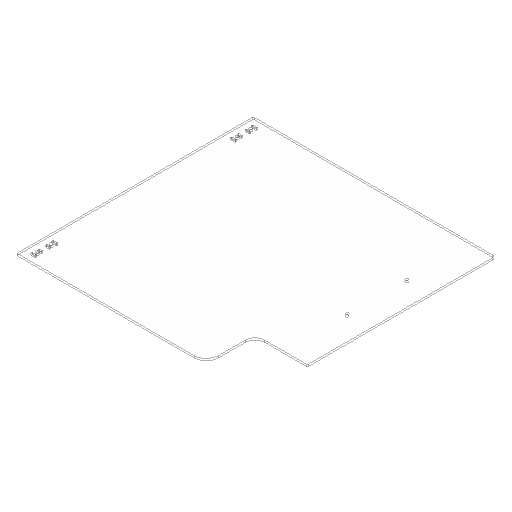
# Autodesk Inventor part: LC_PLEXI_4mm_Front_Door
Saved by Autodesk Inventor 2026.1 (Build 301233000, 233)
## iProperties
Created: 2016-06-27
Part Number: LC_PLEXI_4mm_Front_Door
Material: Ogólny
Document SubType Name: Modeling
Designer: Andrzej
Density: 1 g/cm^3
Appearance: Przezroczysty - jasny
Mass: 916.961 g
Surface Area: 4666.78 cm^2
Volume: 916.961 cm^3
Author: Andrzej
Autodesk Inventor part; units mm, degrees
ref_plane "YZ Plane" through (0, 0, 0) normal (1, 0, 0) x (0, 1, 0)
ref_plane "XZ Plane" through (0, 0, 0) normal (0, 1, 0) x (-1, 0, 0)
ref_plane "XY Plane" through (0, 0, 0) normal (0, 0, 1) x (1, 0, 0)
sketch "Szkic1" plane through (0, 0, 0) normal (0, 0, 1) x (1, 0, 0)
  line L0 (-549.5887, -180.0814) -> (-549.5887, 304.9186)
  line L1 (-549.5887, 304.9186) -> (-53.5887, 304.9186)
  line L2 (-53.5887, 304.9186) -> (-53.5887, -80.0814)
  line L3 (-53.5887, -80.0814) -> (-141.0887, -80.0814)
  line L4 (-161.0887, -100.0814) -> (-161.0887, -155.0814)
  line L5 (-186.0887, -180.0814) -> (-549.5887, -180.0814)
  arc A0 (-141.0887, -80.0814) -> (-161.0887, -100.0814) centre (-141.0887, -100.0814) ccw
  arc A1 (-186.0887, -180.0814) -> (-161.0887, -155.0814) centre (-186.0887, -155.0814) ccw
  point P0 (0, 0)
  point P1 (-161.0887, -80.0814)
  point P2 (-161.0887, -180.0814)
  point P3 (-531.0887, 281.4186)
  point P4 (-531.0887, 253.4186)
  point P5 (-531.0887, -128.5814)
  point P6 (-531.0887, -156.5814)
  point P7 (-103.5887, 173.4186)
  point P8 (-103.5887, 51.4186)
  dimension "d0" = 485
  dimension "d1" = 496
  dimension "d2" = 107.5
  dimension "d3" = 100
  dimension "d6" = 20
  dimension "d7" = 25
  dimension "d8" = 28
  dimension "d9" = 23.5
  dimension "d11" = 28
  dimension "d12" = 23.5
  dimension "d13" = 18.5
  dimension "d14" = 18.5
  dimension "d17" = 18.5
  dimension "d18" = 18.5
  dimension "d31" = 385
  dimension "d32" = 122
  dimension "d33" = 131.5
  dimension "d34" = 50
  dimension "d35" = 50
  constraints: 12 end point, 5 perpendicular, 4 point on circle, 4 point on line, 4 tangent, 2 centre point, 1 vertical
  measures "d0" distance of L0.start L0.end
  measures "d1" distance of L0.end L1.end
  measures "d2" distance between parallel lines of L2 L4
  measures "d3" distance between parallel lines of L5 L3
  measures "d6" radius of A0
  measures "d7" radius of A1
  measures "d8" distance of point (-531.089, 281.419) point (-531.089, 253.419)
  measures "d9" distance from line of L1 point (-531.089, 281.419)
  measures "d11" distance of point (-531.089, -156.581) point (-531.089, -128.581)
  measures "d12" distance from line of L5 point (-531.089, -156.581)
  measures "d13" distance from line of L0 point (-531.089, 281.419)
  measures "d14" distance from line of L0 point (-531.089, 253.419)
  measures "d17" distance from line of L0 point (-531.089, -128.581)
  measures "d18" distance from line of L0 point (-531.089, -156.581)
  measures "d31" distance of L1.end L2.end
  measures "d32" distance of point (-103.589, 173.419) point (-103.589, 51.419)
  measures "d33" distance from line of point (-103.589, 173.419) L1
  measures "d34" distance from line of L2 point (-103.589, 173.419)
  measures "d35" distance from line of L2 point (-103.589, 51.419)
extrude "Wyciągnięcie proste1" add sketch "Szkic1" along normal blind 4
hole "Otwór1" at (-531.0887, 281.4186, 0) at (-531.0887, 253.4186, 0) at (-531.0887, -128.5814, 0) at (-531.0887, -156.5814, 0) direction (0, 0, 1) diameter 6 end through all
fillet "Zaokrąglenie2" radius 2 2 edges at (-53.5887, -80.0814, 2) (-549.5887, -180.0814, 2)
fillet "Zaokrąglenie2" radius 2 1 edges at (-549.5887, 304.9186, 2)
fillet "Zaokrąglenie2" radius 5 1 edges at (-53.5887, 304.9186, 2)
hole "Otwór2" at (-103.5887, 173.4186, 0) at (-103.5887, 51.4186, 0) direction (0, 0, 1) diameter 6 end through all
sketch "Szkic2" plane through (0, 0, 4) normal (0, 0, 1) x (1, 0, 0)
  circle A0 centre (-103.5887, 173.4186) radius 3 projected
  circle A1 centre (-103.5887, 51.4186) radius 3 projected
  arc A2 (-53.5887, 299.9186) -> (-58.5887, 304.9186) centre (-58.5887, 299.9186) ccw projected
  line L0 (-58.5887, 304.9186) -> (-547.5887, 304.9186) projected
  arc A3 (-547.5887, 304.9186) -> (-549.5887, 302.9186) centre (-547.5887, 302.9186) ccw projected
  line L1 (-549.5887, 302.9186) -> (-549.5887, -178.0814) projected
  arc A4 (-549.5887, -178.0814) -> (-547.5887, -180.0814) centre (-547.5887, -178.0814) ccw projected
  line L2 (-547.5887, -180.0814) -> (-186.0887, -180.0814) projected
  arc A5 (-186.0887, -180.0814) -> (-161.0887, -155.0814) centre (-186.0887, -155.0814) ccw projected
  line L3 (-161.0887, -155.0814) -> (-161.0887, -100.0814) projected
  arc A6 (-141.0887, -80.0814) -> (-161.0887, -100.0814) centre (-141.0887, -100.0814) ccw projected
  line L4 (-141.0887, -80.0814) -> (-55.5887, -80.0814) projected
  arc A7 (-55.5887, -80.0814) -> (-53.5887, -78.0814) centre (-55.5887, -78.0814) ccw projected
  line L5 (-53.5887, -78.0814) -> (-53.5887, 299.9186) projected
  circle A8 centre (-531.0887, -128.5814) radius 3 projected
  circle A9 centre (-531.0887, 281.4186) radius 3 projected
  circle A10 centre (-531.0887, 253.4186) radius 3 projected
  circle A11 centre (-531.0887, -156.5814) radius 3 projected
  line L6 (-535.1387, 289.5186) -> (-527.0387, 289.5186)
  line L7 (-527.0387, 289.5186) -> (-527.0387, 288.1686)
  line L8 (-527.0387, 288.1686) -> (-535.1387, 288.1686)
  line L9 (-535.1387, 288.1686) -> (-535.1387, 289.5186)
  line L10 (-534.1387, 276.1686) -> (-528.0387, 276.1686)
  line L11 (-528.0387, 276.1686) -> (-528.0387, 274.8186)
  line L12 (-528.0387, 274.8186) -> (-534.1387, 274.8186)
  line L13 (-534.1387, 274.8186) -> (-534.1387, 276.1686)
  line L14 (-534.1387, 260.0186) -> (-528.0387, 260.0186)
  line L15 (-528.0387, 260.0186) -> (-528.0387, 258.6686)
  line L16 (-528.0387, 258.6686) -> (-534.1387, 258.6686)
  line L17 (-534.1387, 258.6686) -> (-534.1387, 260.0186)
  line L18 (-535.1387, 245.3186) -> (-527.0387, 245.3186)
  line L19 (-527.0387, 245.3186) -> (-527.0387, 246.6686)
  line L20 (-527.0387, 246.6686) -> (-535.1387, 246.6686)
  line L21 (-535.1387, 246.6686) -> (-535.1387, 245.3186)
  line L22 (-535.6387, 287.6686) -> (-526.5387, 287.6686)
  line L23 (-526.5387, 287.6686) -> (-526.5387, 290.0186)
  line L24 (-526.5387, 290.0186) -> (-535.6387, 290.0186)
  line L25 (-535.6387, 290.0186) -> (-535.6387, 287.6686)
  line L26 (-534.6387, 274.3186) -> (-527.5387, 274.3186)
  line L27 (-527.5387, 274.3186) -> (-527.5387, 276.6686)
  line L28 (-527.5387, 276.6686) -> (-534.6387, 276.6686)
  line L29 (-534.6387, 276.6686) -> (-534.6387, 274.3186)
  line L30 (-534.6387, 258.1686) -> (-527.5387, 258.1686)
  line L31 (-527.5387, 258.1686) -> (-527.5387, 260.5186)
  line L32 (-527.5387, 260.5186) -> (-534.6387, 260.5186)
  line L33 (-534.6387, 260.5186) -> (-534.6387, 258.1686)
  line L34 (-535.6387, 247.1686) -> (-526.5387, 247.1686)
  line L35 (-526.5387, 247.1686) -> (-526.5387, 244.8186)
  line L36 (-526.5387, 244.8186) -> (-535.6387, 244.8186)
  line L37 (-535.6387, 244.8186) -> (-535.6387, 247.1686)
  line L38 (-535.1387, -120.4814) -> (-527.0387, -120.4814)
  line L39 (-527.0387, -120.4814) -> (-527.0387, -121.8314)
  line L40 (-527.0387, -121.8314) -> (-535.1387, -121.8314)
  line L41 (-535.1387, -121.8314) -> (-535.1387, -120.4814)
  line L42 (-534.1387, -133.8314) -> (-528.0387, -133.8314)
  line L43 (-528.0387, -133.8314) -> (-528.0387, -135.1814)
  line L44 (-528.0387, -135.1814) -> (-534.1387, -135.1814)
  line L45 (-534.1387, -135.1814) -> (-534.1387, -133.8314)
  line L46 (-534.1387, -149.9814) -> (-528.0387, -149.9814)
  line L47 (-528.0387, -149.9814) -> (-528.0387, -151.3314)
  line L48 (-528.0387, -151.3314) -> (-534.1387, -151.3314)
  line L49 (-534.1387, -151.3314) -> (-534.1387, -149.9814)
  line L50 (-535.1387, -164.6814) -> (-527.0387, -164.6814)
  line L51 (-527.0387, -164.6814) -> (-527.0387, -163.3314)
  line L52 (-527.0387, -163.3314) -> (-535.1387, -163.3314)
  line L53 (-535.1387, -163.3314) -> (-535.1387, -164.6814)
  line L54 (-535.6387, -122.3314) -> (-526.5387, -122.3314)
  line L55 (-526.5387, -122.3314) -> (-526.5387, -119.9814)
  line L56 (-526.5387, -119.9814) -> (-535.6387, -119.9814)
  line L57 (-535.6387, -119.9814) -> (-535.6387, -122.3314)
  line L58 (-534.6387, -135.6814) -> (-527.5387, -135.6814)
  line L59 (-527.5387, -135.6814) -> (-527.5387, -133.3314)
  line L60 (-527.5387, -133.3314) -> (-534.6387, -133.3314)
  line L61 (-534.6387, -133.3314) -> (-534.6387, -135.6814)
  line L62 (-534.6387, -151.8314) -> (-527.5387, -151.8314)
  line L63 (-527.5387, -151.8314) -> (-527.5387, -149.4814)
  line L64 (-527.5387, -149.4814) -> (-534.6387, -149.4814)
  line L65 (-534.6387, -149.4814) -> (-534.6387, -151.8314)
  line L66 (-535.6387, -162.8314) -> (-526.5387, -162.8314)
  line L67 (-526.5387, -162.8314) -> (-526.5387, -165.1814)
  line L68 (-526.5387, -165.1814) -> (-535.6387, -165.1814)
  line L69 (-535.6387, -165.1814) -> (-535.6387, -162.8314)
  point P0 (0, 0)
  dimension "d43" = 8.1
  dimension "d44" = 1.35
  dimension "d45" = 6.1
  dimension "d46" = 1.35
  dimension "d47" = 6.1
  dimension "d48" = 1.35
  dimension "d49" = 8.1
  dimension "d50" = 1.35
  dimension "d51" = 4.05
  dimension "d52" = 3.05
  dimension "d53" = 3.05
  dimension "d54" = 4.05
  dimension "d55" = 8.1
  dimension "d56" = 8.1
  dimension "d57" = 6.6
  dimension "d59" = 44.2
  dimension "d60" = 17.5
  dimension "d61" = 14.8
  dimension "d62" = 6.6
  dimension "d63" = 0.5
  dimension "d64" = 0.5
  dimension "d65" = 0.5
  dimension "d66" = 0.5
  dimension "d69" = 8.1
  dimension "d70" = 1.35
  dimension "d71" = 6.1
  dimension "d72" = 1.35
  dimension "d73" = 6.1
  dimension "d74" = 1.35
  dimension "d75" = 8.1
  dimension "d76" = 1.35
  dimension "d77" = 44.2
  dimension "d78" = 17.5
  dimension "d79" = 14.8
  dimension "d80" = 0.5
  dimension "d81" = 0.5
  dimension "d82" = 0.5
  dimension "d83" = 0.5
  dimension "d84" = 8.1
  dimension "d85" = 6.6
  dimension "d86" = 6.6
  dimension "d87" = 8.1
  dimension "d88" = 3.05
  dimension "d89" = 4.05
  dimension "d90" = 4.05
  dimension "d91" = 3.05
  constraints: 128 end point, 32 parallel, 16 perpendicular, 8 horizontal, 24 other
  measures "d43" distance of L7.end L8.end
  measures "d44" distance of L6.end L7.end
  measures "d45" distance of L11.end L12.end
  measures "d46" distance of L10.end L11.end
  measures "d47" distance of L15.end L16.end
  measures "d48" distance of L14.end L15.end
  measures "d49" distance of L20.end L19.end
  measures "d50" distance of L19.end L18.end
  measures "d51" distance from line of A9.centre L9
  measures "d52" distance from line of A9.centre L13
  measures "d53" distance from line of L17 A10.centre
  measures "d54" distance from line of L21 A10.centre
  measures "d55" distance from line of L6 A9.centre
  measures "d56" distance from line of A10.centre L18
  measures "d57" distance from line of A9.centre L12
  measures "d59" distance between parallel lines of L18 L6
  measures "d60" distance between parallel lines of L16 L10
  measures "d61" distance between parallel lines of L14 L12
  measures "d62" distance from line of L14 A10.centre
  measures "d63" distance between parallel lines of L8 L22
  measures "d64" distance between parallel lines of L12 L26
  measures "d65" distance between parallel lines of L16 L30
  measures "d66" distance between parallel lines of L20 L34
  measures "d69" distance of L40.start L40.end
  measures "d70" distance of L39.start L40.start
  measures "d71" distance of L44.start L45.start
  measures "d72" distance of L42.end L44.start
  measures "d73" distance of L47.end L48.end
  measures "d74" distance of L47.start L47.end
  measures "d75" distance of L52.end L52.start
  measures "d76" distance of L52.start L50.end
  measures "d77" distance between parallel lines of L50 L38
  measures "d78" distance between parallel lines of L48 L42
  measures "d79" distance between parallel lines of L46 L44
  measures "d80" distance between parallel lines of L40 L54
  measures "d81" distance between parallel lines of L44 L58
  measures "d82" distance between parallel lines of L48 L62
  measures "d83" distance between parallel lines of L52 L66
  measures "d84" distance from line of L38 A8.centre
  measures "d85" distance from line of L44 A8.centre
  measures "d86" distance from line of A11.centre L46
  measures "d87" distance from line of A11.centre L50
  measures "d88" distance from line of A11.centre L49
  measures "d89" distance from line of A11.centre L53
  measures "d90" distance from line of A8.centre L41
  measures "d91" distance from line of A8.centre L45
extrude "Wyciągnięcie proste2" cut sketch "Szkic2" against normal through all contours L6 L7 L8 L9 | L10 L11 L12 L13 | L14 L15 L16 L17 | L21 L20 L19 L18 | L25 L24 L23 L22 | L29 L28 L27 L26 | L33 L32 L31 L30 | L34 L35 L36 L37 | L38 L39 L40 L41 | L42 L43 L44 L45 | L46 L47 L48 L49 | L53 L52 L51 L50 | L57 L56 L55 L54 | L61 L60 L59 L58 | L65 L64 L63 L62 | L66 L67 L68 L69
equation "\"d11\" = d8"
equation "\"d12\" = d9"
equation "\"d14\" = d13"
equation "\"d17\" = d13"
equation "\"d18\" = d13"
equation "\"d33\" = -0.5 * d32 + 0.5 * d31"
equation "\"d34\" = d35"
equation "\"d51\" = 0.5 * d43"
equation "\"d52\" = 0.5 * d45"
equation "\"d53\" = 0.5 * d47"
equation "\"d54\" = 0.5 * d49"
equation "\"d64\" = d63"
equation "\"d65\" = d63"
equation "\"d66\" = d63"
equation "\"d80\" = d63"
equation "\"d81\" = d80"
equation "\"d82\" = d80"
equation "\"d83\" = d80"
